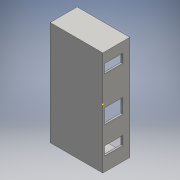
# Autodesk Inventor part: Pièce
Saved by Autodesk Inventor 2016 SP1 (Build 200210100, 210)
## iProperties
Created: 2016-10-04
Part Number: Pièce
Material: Générique
Document SubType Name: Modeling
Designer: dimercur
Density: 1 g/cm^3
Appearance: Par défaut
Author: dimercur
Autodesk Inventor part; units mm, degrees
ref_plane "YZ Plane" through (0, 0, 0) normal (1, 0, 0) x (0, 1, 0)
ref_plane "XZ Plane" through (0, 0, 0) normal (0, 1, 0) x (-1, 0, 0)
ref_plane "XY Plane" through (0, 0, 0) normal (0, 0, 1) x (1, 0, 0)
sketch "Esquisse1" plane through (0, 0, 0) normal (0, 1, 0) x (-1, 0, 0)
  line L0 (2364.0452, 5297.7399) -> (-3875.9548, 5297.7399)
  line L1 (-3875.9548, 5297.7399) -> (-3875.9548, -7052.2601)
  line L2 (-3875.9548, -7052.2601) -> (2364.0452, -7052.2601)
  line L3 (2364.0452, -7052.2601) -> (2364.0452, 5297.7399)
  point P0 (0, 0)
  dimension "d0" = 12350
  dimension "d1" = 6240
  constraints: 8 end point, 2 parallel, 1 horizontal, 1 perpendicular
  measures "d0" distance of L2.end L0.start
  measures "d1" distance of L0.start L0.end
extrude "Extrusion1" add sketch "Esquisse1" along normal blind 3200
shell "Coque1" thickness 200 removed faces 1 at (-284.0452, 3200, 1181.0732)
sketch "Esquisse2" plane through (3875.9548, 0, 5297.7399) normal (1, 0, 0) x (0, 0, -1)
  line L0 (200, 200) -> (12150, 200) projected
  line L1 (5750, 2350) -> (7470, 2350)
  line L2 (7470, 2350) -> (7470, 200)
  line L3 (7470, 200) -> (5750, 200)
  line L4 (5750, 200) -> (5750, 2350)
  line L5 (9650, 2350) -> (10700, 2350)
  line L6 (10700, 2350) -> (10700, 200)
  line L7 (10700, 200) -> (9650, 200)
  line L8 (9650, 200) -> (9650, 2350)
  line L9 (12150, 200) -> (12150, 3200) projected
  line L10 (1200, 2350) -> (2250, 2350)
  line L11 (2250, 2350) -> (2250, 200)
  line L12 (2250, 200) -> (1200, 200)
  line L13 (1200, 200) -> (1200, 2350)
  line L14 (200, 200) -> (200, 3200) projected
  point P0 (5297.7399, 0)
  dimension "d5" = 1050
  dimension "d6" = 1450
  dimension "d7" = 2150
  dimension "d8" = 1720
  dimension "d10" = 4680
  dimension "d32" = 1050
  dimension "d33" = 1000
  dimension "d34" = 2150
  constraints: 24 end point, 6 parallel, 4 point on line, 3 horizontal, 3 perpendicular
  measures "d5" distance between parallel lines of L6 L8
  measures "d6" distance between parallel lines of L9 L6
  measures "d7" distance of L7.end L5.start
  measures "d8" distance between parallel lines of L2 L4
  measures "d10" distance between parallel lines of L9 L2
  measures "d32" distance of L10.start L10.end
  measures "d33" distance between parallel lines of L14 L13
  measures "d34" distance between parallel lines of L0 L10
extrude "Extrusion2" cut sketch "Esquisse2" against normal blind 3000
sketch "Esquisse3" plane through (-2364.0452, 0, -7052.2601) normal (-1, 0, 0) x (0, 0, 1)
  line L0 (325, 3000) -> (1825, 3000)
  line L1 (1825, 3000) -> (1825, 1100)
  line L2 (1825, 1100) -> (325, 1100)
  line L3 (325, 1100) -> (325, 3000)
  line L4 (200, 200) -> (12150, 200) projected
  line L5 (200, 200) -> (200, 3200) projected
  point P0 (7052.2601, 0)
  dimension "d13" = 900
  dimension "d14" = 1900
  dimension "d15" = 1500
  dimension "d16" = 125
  constraints: 8 end point, 2 parallel, 1 horizontal, 1 perpendicular
  measures "d13" distance from line of L4 L2.end
  measures "d14" distance of L2.end L0.start
  measures "d15" distance between parallel lines of L1 L3
  measures "d16" distance between parallel lines of L5 L3
extrude "Extrusion3" cut sketch "Esquisse3" against normal blind 3000
pattern_linear "Réseau rectangulaire1" count 7 spacing 1700 along (0, 0, 1) of "Extrusion3"
sketch "Esquisse4" plane through (-2164.0452, 200, -6852.2601) normal (0, 1, 0) x (1, 0, 0)
  line L0 (530, -3310) -> (230, -3310)
  line L1 (230, -3310) -> (230, -3540)
  line L2 (230, -3540) -> (530, -3540)
  line L3 (530, -3540) -> (530, -3310)
  line L4 (0, 0) -> (5840, 0) projected
  line L5 (0, -11950) -> (0, 0) projected
  point P0 (2164.0452, -6852.2601)
  dimension "d22" = 230
  dimension "d23" = 300
  dimension "d25" = 3540
  dimension "d26" = 230
  constraints: 8 end point, 2 parallel, 1 horizontal, 1 perpendicular
  measures "d22" distance of L2.end L0.start
  measures "d23" distance of L1.end L2.end
  measures "d25" distance between parallel lines of L4 L2
  measures "d26" distance between parallel lines of L5 L1
extrude "Extrusion4" add sketch "Esquisse4" along normal blind 3000
pattern_linear "Réseau rectangulaire2" count 3 spacing 3390 along (0, 0, 1) of "Extrusion4"
sketch "Esquisse5" plane through (3875.9548, 0, 5297.7399) normal (1, 0, 0) x (0, 0, -1)
  point P0 (5297.7399, 0)
